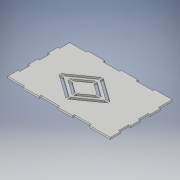
# Autodesk Inventor part: ATAS
Saved by Autodesk Inventor 2019 (Build 230136000, 136)
## iProperties
Created: 2019-11-24
Part Number: ATAS
Material: Generic
Document SubType Name: Modeling
Designer: User
Density: 1 g/cm^3
Appearance: Default
Author: User
Autodesk Inventor part; units mm, degrees
ref_plane "YZ Plane" through (0, 0, 0) normal (1, 0, 0) x (0, 1, 0)
ref_plane "XZ Plane" through (0, 0, 0) normal (0, 1, 0) x (-1, 0, 0)
ref_plane "XY Plane" through (0, 0, 0) normal (0, 0, 1) x (1, 0, 0)
sketch "Sketch1" plane through (0, 0, 0) normal (0, 1, 0) x (-1, 0, 0)
  line L0 (-55.3, 34) -> (55.3, -34) construction
  line L1 (55.3424, 32) -> (55.3424, 21)
  line L2 (53.3, 10) -> (55.3, 10)
  line L3 (55.3, 10) -> (55.3, -1)
  line L4 (55.3, -1) -> (53.3, -1)
  line L5 (53.3, -1) -> (53.3, -12)
  line L6 (53.3, -12) -> (55.3, -12)
  line L7 (55.3, -12) -> (55.3, -23)
  line L8 (55.3, -23) -> (53.3, -23)
  line L9 (55.3424, 21) -> (55.3424, 32)
  line L10 (55.3, -23) -> (55.3, -12)
  line L11 (55.3, -1) -> (55.3, 10)
  line L12 (-53.3, 0.4465) -> (-53.3, 0.446)
  line L13 (-53.3487, -21) -> (-53.3, -21)
  line L14 (55.3424, 32) -> (37.0424, 32)
  line L15 (37.0424, 32) -> (37.0424, 34)
  line L16 (37.0424, 34) -> (18.7424, 34)
  line L17 (18.7424, 34) -> (18.7424, 32)
  line L18 (18.7424, 32) -> (-1.6, 32)
  line L19 (-1.6, 32) -> (-1.6, 34)
  line L20 (-1.6, 34) -> (-17.9, 34)
  line L21 (-17.9, 34) -> (-17.9, 32)
  line L22 (-17.9, 32) -> (-36.2, 32)
  line L23 (-36.2, 32) -> (-36.2, 34)
  line L24 (37.0424, 34) -> (18.7424, 34)
  line L25 (-1.6, 34) -> (-17.9, 34)
  line L26 (-36.2, 34) -> (-55.3, 34)
  line L27 (2.5632, 10.7554) -> (14.3549, 2.3144)
  line L28 (0.7434, 10.7554) -> (-11.0739, 2.3144)
  line L29 (19.1722, 2.3144) -> (2.5632, 14.178)
  line L30 (0.7434, 14.1963) -> (-15.8912, 2.3144)
  line L31 (-20.6639, 0.446) -> (0.7434, -14.8449)
  line L32 (2.5632, -14.8267) -> (23.9449, 0.446)
  line L33 (23.9895, 2.3144) -> (2.5632, 17.6189)
  line L34 (0.7434, 17.6372) -> (-20.7085, 2.3144)
  line L35 (-25.4812, 0.446) -> (0.7434, -18.2859)
  line L36 (2.5632, -18.2676) -> (28.7623, 0.446)
  line L37 (28.8068, 2.3144) -> (2.5632, 21.0599)
  line L38 (41.2856, 32.5499) -> (41.2856, 32.5817)
  line L39 (54.8971, 24.1408) -> (54.9227, 24.1408)
  line L40 (14.3549, 0.446) -> (14.3549, 0.4779)
  line L41 (0.7434, 21.0782) -> (-25.5258, 2.3144)
  line L42 (-11.0739, 2.3144) -> (-15.8912, 2.3144)
  line L43 (-20.7085, 2.3144) -> (-25.5258, 2.3144)
  line L44 (0.7434, 21.0782) -> (0.7434, 17.6372)
  line L45 (0.7434, 14.1963) -> (0.7434, 10.7554)
  line L46 (2.5632, 10.7554) -> (2.5632, 14.178)
  line L47 (2.5632, 17.6189) -> (2.5632, 21.0599)
  line L48 (14.3549, 2.3144) -> (19.1722, 2.3144)
  line L49 (23.9895, 2.3144) -> (28.8068, 2.3144)
  line L50 (28.7623, 0.446) -> (23.9449, 0.446)
  line L51 (2.5632, -14.8267) -> (2.5632, -18.2676)
  line L52 (0.7434, -18.2859) -> (0.7434, -14.8449)
  line L53 (-25.4812, 0.446) -> (-20.6639, 0.446)
  line L54 (-11.0739, 0.4464) -> (-15.8912, 0.4464)
  line L55 (0.7434, -7.9945) -> (-11.0739, 0.4464)
  line L56 (0.7434, -11.4354) -> (-15.8912, 0.4464)
  line L57 (0.7434, -11.4354) -> (0.7434, -7.9945)
  line L58 (-11.7935, 1.3804) -> (-5.9618, 1.3804)
  line L59 (2.5632, 10.7554) -> (2.5632, 10.7554)
  line L60 (2.5632, -7.9945) -> (2.5632, -11.4171)
  line L61 (14.3549, 0.4464) -> (19.1722, 0.4464)
  line L62 (19.1722, 0.4464) -> (2.5632, -11.4171)
  line L63 (2.5632, -7.9945) -> (14.3549, 0.4464)
  line L64 (19.1722, 0.4464) -> (14.3549, 0.4464)
  line L65 (14.3549, 0.4464) -> (2.5632, -7.9945)
  line L66 (2.5632, -7.9945) -> (2.5632, -11.4171)
  line L67 (2.5632, -11.4171) -> (19.1722, 0.4464)
  line L68 (53.3, 10) -> (53.3, 21)
  line L69 (53.3, 21) -> (55.3424, 21)
  line L70 (53.3, -34.0004) -> (53.3, -34.0004)
  line L71 (53.3, -23) -> (53.3, -32)
  line L72 (34.2, -32.0004) -> (34.2, -32)
  line L73 (55.3, 34) -> (-52.0471, -32) construction
  line L74 (53.3, -32) -> (53.3, -34.0004)
  line L75 (-39, -36.0004) -> (-53.3, -36.0004)
  line L76 (-53.3, -36.0004) -> (-57.3, -36.0004)
  line L77 (-57.3, -36.0004) -> (-57.3, -21.0004)
  line L78 (-57.3, -21.0004) -> (-59.3, -21.0004)
  line L79 (-59.3, -21.0004) -> (-59.3, -9.7058)
  line L80 (-59.3, -9.7058) -> (-57.3, -9.7058)
  line L81 (-57.3, -9.7058) -> (-57.3, 0.4464)
  line L82 (-57.3, 0.4464) -> (-57.3, 1)
  line L83 (-57.3, 1) -> (-59.3, 1)
  line L84 (-59.3, 1) -> (-59.3, 12)
  line L85 (-59.3, 12) -> (-57.3, 12)
  line L86 (-57.3, 12) -> (-57.3, 23)
  line L87 (-57.3, 23) -> (-59.3, 23)
  line L88 (-59.3, 23) -> (-59.3, 34)
  line L89 (-59.3, 34) -> (-55.3, 34)
  line L90 (-53.3, -21) -> (-53.3, -21.0004)
  line L91 (-55.3, 32.0365) -> (-55.3, 32)
  line L92 (-55.3, 32.0365) -> (-55.3, 32)
  line L93 (-39, -36.0004) -> (-38.1942, -36.0004)
  line L94 (53.3, -34.0004) -> (35, -34.0004)
  line L95 (35, -34.0004) -> (35, -36.0004)
  line L96 (35, -36.0004) -> (18.7, -36.0004)
  line L97 (18.7, -36.0004) -> (16.7, -36.0004)
  line L98 (16.7, -36.0004) -> (16.7, -34.0004)
  line L99 (16.7, -34.0004) -> (-1.6, -34.0004)
  line L100 (-1.6, -34.0004) -> (-1.6, -36.0004)
  line L101 (-1.6, -36.0004) -> (-17.9, -36.0004)
  line L102 (-17.9, -36.0004) -> (-19.9, -36.0004)
  line L103 (-19.9, -36.0004) -> (-19.9, -34.0004)
  line L104 (-19.9, -34.0004) -> (-38.2, -34.0004)
  line L105 (-38.2, -34.0004) -> (-38.1942, -36.0004)
  point P0 (0, 0)
  point P1 (-53.3, 20.3166)
  point P2 (-53.3, 1)
  point P3 (-53.3, -10)
  point P4 (-55.3, -18.9529)
  point P5 (-53.3, -32.7703)
  point P6 (-16.7, -32.027)
  point P7 (-21.4801, -32.0004)
  point P8 (-17.9, -36.0004)
  dimension "d30" = 1.868
  dimension "d31" = 0.934
  dimension "d34" = 11
  dimension "d35" = 11
  dimension "d36" = 11
  dimension "d37" = 11
  dimension "d38" = 11
  dimension "d61" = 4
  dimension "d70" = 18.3
  dimension "d72" = 2
  dimension "d73" = 18.3
  dimension "d75" = 2
  constraints: 212 end point, 42 perpendicular, 21 point on line, 14 horizontal, 11 parallel, 6 vertical, 5 symmetric about line, 4 collinear, 1 midpoint
  measures "d30" distance between parallel lines of L42 L54
  measures "d31" distance between parallel lines of L54 L58
  measures "d34" distance of L1.start L1.end
  measures "d35" distance of L2.end L3.end
  measures "d36" distance of L6.end L7.end
  measures "d37" distance of L2.start L68.end
  measures "d38" distance of L4.end L5.end
  measures "d61" distance of L75.end L76.end
  measures "d70" distance of L70.start L94.end
  measures "d72" distance of L96.end L97.end
  measures "d73" distance of L98.end L99.end
  measures "d75" distance of L101.end L102.end
extrude "Extrusion1" add sketch "Sketch1" along normal blind 2
body "Solid1"
